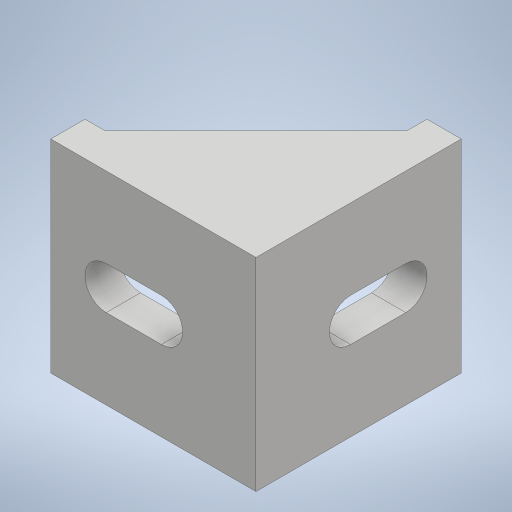
# Autodesk Inventor part: escuadra pequeña
Saved by Autodesk Inventor 2024.2 (Build 282272000, 272)
## iProperties
Created: 2025-07-02
Part Number: escuadra pequeña
Material: Genérico
Document SubType Name: Modeling
Designer: jd.castellanosq
Density: 1 g/cm^3
Appearance: Valor por defecto
Author: jd.castellanosq
Autodesk Inventor part; units mm, degrees
ref_plane "YZ Plane" through (0, 0, 0) normal (1, 0, 0) x (0, 1, 0)
ref_plane "XZ Plane" through (0, 0, 0) normal (0, 1, 0) x (-1, 0, 0)
ref_plane "XY Plane" through (0, 0, 0) normal (0, 0, 1) x (1, 0, 0)
sketch "Boceto1" plane through (0, 0, 0) normal (0, 0, 1) x (1, 0, 0)
  line L0 (0, 0) -> (42, 0)
  line L1 (42, 0) -> (42, 42)
  line L2 (42, 42) -> (35, 42)
  line L3 (35, 42) -> (35, 7)
  line L4 (35, 7) -> (0, 7)
  line L5 (0, 7) -> (0, 0)
  dimension "d0" = 7
  dimension "d1" = 7
  dimension "d2" = 42
  dimension "d3" = 42
  constraints: 12 end point, 5 perpendicular, 1 horizontal
  measures "d0" distance between parallel lines of L4 L0
  measures "d1" distance between parallel lines of L1 L3
  measures "d2" distance of L0.start L0.end
  measures "d3" distance of L0.end L1.end
extrude "Extrusión1" add sketch "Boceto1" along normal blind 41.5
sketch "Boceto2" plane through (0, 0, 41.5) normal (0, 0, 1) x (1, 0, 0)
  line L0 (35, 7) -> (0, 7) projected
  line L1 (35, 7) -> (35, 38)
  line L2 (35, 42) -> (35, 7) projected
  line L3 (35, 38) -> (4, 7)
  line L4 (4, 7) -> (35, 7)
  line L5 (42, 42) -> (35, 42) projected
  point P0 (0, 0)
  point P1 (4, 7)
  dimension "d6" = 4
  dimension "d7" = 4
  constraints: 6 end point, 1 perpendicular, 1 point on line
  measures "d6" distance from line of L5 L1.end
  measures "d7" distance of L3.end L0.end
extrude "Extrusión2" add sketch "Boceto2" against normal blind 4
sketch "Boceto3" plane through (0, 0, 0) normal (0, 0, -1) x (-1, 0, 0)
  line L0 (-4, 7) -> (-35, 38) projected
  line L1 (-35, 42) -> (-35, 7) projected
  line L2 (-35, 7) -> (0, 7) projected
  point P0 (0, 0)
extrude "Extrusión3" add sketch "Boceto3" against normal blind 4
sketch "Boceto4" plane through (35, 42, 0) normal (-1, 0, 0) x (0, 0, 1)
  line L0 (20.75, -11.35) -> (20.75, -22.65) construction
  line L1 (16.4, -11.35) -> (16.4, -22.65)
  line L2 (25.1, -22.65) -> (25.1, -11.35)
  arc A0 (25.1, -11.35) -> (16.4, -11.35) centre (20.75, -11.35) ccw
  arc A1 (16.4, -22.65) -> (25.1, -22.65) centre (20.75, -22.65) ccw
  line L3 (0, 0) -> (41.5, 0) projected
  point P0 (0, -42)
  point P1 (20.75, -17)
  point P2 (20.75, 0)
  point P3 (20.75, -27)
  point P4 (20.75, -7)
  dimension "d12" = 8.7
  dimension "d13" = 20
  dimension "d14" = 7
  constraints: 8 end point, 6 point on circle, 4 tangent, 2 centre point, 2 midpoint, 1 parallel, 1 vertical, 1 vertical alignment
  measures "d12" distance between parallel lines of L2 L1
  measures "d13" distance of point (20.75, -27) point (20.75, -7)
  measures "d14" distance from line of L3 point (20.75, -7)
extrude "Extrusión4" cut sketch "Boceto4" against normal through all
sketch "Boceto5" plane through (0, 7, 41.5) normal (0, 1, 0) x (1, 0, 0)
  line L0 (22.65, 20.75) -> (11.35, 20.75) construction
  line L1 (22.65, 25.1) -> (11.35, 25.1)
  line L2 (11.35, 16.4) -> (22.65, 16.4)
  arc A0 (22.65, 16.4) -> (22.65, 25.1) centre (22.65, 20.75) ccw
  arc A1 (11.35, 25.1) -> (11.35, 16.4) centre (11.35, 20.75) ccw
  line L3 (0, 41.5) -> (0, 0) projected
  point P0 (17, 20.75)
  point P1 (0, 20.75)
  point P2 (27, 20.75)
  point P3 (7, 20.75)
  dimension "d17" = 20
  dimension "d18" = 7
  dimension "d19" = 8.7
  constraints: 8 end point, 6 point on circle, 4 tangent, 2 centre point, 2 midpoint, 1 horizontal, 1 horizontal alignment, 1 parallel
  measures "d17" distance of point (27, 20.75) point (7, 20.75)
  measures "d18" distance from line of L3 point (7, 20.75)
  measures "d19" distance between parallel lines of L2 L1
extrude "Extrusión5" cut sketch "Boceto5" against normal blind 10
